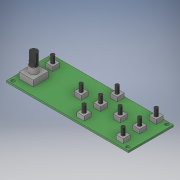
# Autodesk Inventor part: Keypad
Saved by Autodesk Inventor 2018 (Build 220112000, 112)
## iProperties
Created: 2013-10-28
Part Number: Keypad
Material: Generic
Document SubType Name: Modeling
Designer: Gabriel Smolnycki
Mass: 8.54171 g
Surface Area: 100.523 cm^2
Volume: 8.54171 cm^3
Density: 1 g/cm^3
Appearance: Default
Sending System: SolidWorks 2017
Last Author: Gabriel Smolnycki
Last Saved: 2017-09-14
Author: Gabriel Smolnycki
Autodesk Inventor part; units mm, degrees
ref_plane "YZ Plane" through (0, 0, 0) normal (1, 0, 0) x (0, 1, 0)
ref_plane "XZ Plane" through (0, 0, 0) normal (0, 1, 0) x (-1, 0, 0)
ref_plane "XY Plane" through (0, 0, 0) normal (0, 0, 1) x (1, 0, 0)
sketch "Sketch1" plane through (0, 0, 0) normal (0, 1, 0) x (-1, 0, 0)
  line L0 (-51.5, -19) -> (51.5, -19)
  line L1 (-51.5, 19) -> (-51.5, -19)
  line L2 (51.5, 19) -> (-51.5, 19)
  line L3 (51.5, -19) -> (51.5, 19)
  constraints: 8 end point, 2 horizontal, 2 vertical
extrude "Extrusion23" add sketch "Sketch1" along normal blind 1.5
hole "Hole4" at (48.5, 0, -16.5) direction (0, 1, 0) diameter 3 depth 1.5
hole "Hole3" at (48.5, 0, 16.5) direction (0, 1, 0) diameter 3 depth 1.5
sketch "Sketch3" plane through (0, 0, 0) normal (0, 1, 0) x (-1, 0, 0)
  point P0 (-48.5, 16.5)
hole "Hole2" at (-48.5, 0, 16.5) direction (0, 1, 0) diameter 3 depth 1.5
sketch "Sketch2" plane through (0, 0, 0) normal (0, 1, 0) x (-1, 0, 0)
  point P0 (-48.5, -16.5)
hole "Hole1" at (-48.5, 0, -16.5) direction (0, 1, 0) diameter 3 depth 1.5
sketch "Sketch6" plane through (0, 1.5, 0) normal (0, 1, 0) x (1, 0, 0)
  line L0 (44, 18) -> (38, 18)
  line L1 (44, 12) -> (44, 18)
  line L2 (38, 12) -> (44, 12)
  line L3 (38, 18) -> (38, 12)
  constraints: 8 end point, 2 horizontal, 2 vertical, 1 perpendicular
extrude "Extrusion22" add sketch "Sketch6" along normal blind 3.5
sketch "Sketch7" plane through (0, 1.5, 0) normal (0, 1, 0) x (1, 0, 0)
  line L0 (38, 4) -> (38, -2)
  line L1 (44, 4) -> (38, 4)
  line L2 (44, -2) -> (44, 4)
  line L3 (38, -2) -> (44, -2)
  constraints: 8 end point, 2 horizontal, 2 vertical, 1 perpendicular
extrude "Extrusion21" add sketch "Sketch7" along normal blind 3.5
sketch "Sketch8" plane through (0, 1.5, 0) normal (0, 1, 0) x (1, 0, 0)
  line L0 (38, -16) -> (44, -16)
  line L1 (38, -10) -> (38, -16)
  line L2 (44, -10) -> (38, -10)
  line L3 (44, -16) -> (44, -10)
  constraints: 8 end point, 2 horizontal, 2 vertical, 1 perpendicular
extrude "Extrusion20" add sketch "Sketch8" along normal blind 3.5
sketch "Sketch9" plane through (0, 1.5, 0) normal (0, 1, 0) x (1, 0, 0)
  line L0 (27.5, -2) -> (27.5, 4)
  line L1 (21.5, -2) -> (27.5, -2)
  line L2 (27.5, 4) -> (21.5, 4)
  line L3 (21.5, 4) -> (21.5, -2)
  constraints: 8 end point, 2 horizontal, 2 vertical, 1 perpendicular
extrude "Extrusion19" add sketch "Sketch9" along normal blind 3.5
sketch "Sketch10" plane through (0, 1.5, 0) normal (0, 1, 0) x (1, 0, 0)
  line L0 (5, 18) -> (5, 12)
  line L1 (11, 18) -> (5, 18)
  line L2 (11, 12) -> (11, 18)
  line L3 (5, 12) -> (11, 12)
  constraints: 8 end point, 2 horizontal, 2 vertical, 1 perpendicular
extrude "Extrusion18" add sketch "Sketch10" along normal blind 3.5
sketch "Sketch11" plane through (0, 1.5, 0) normal (0, 1, 0) x (1, 0, 0)
  line L0 (11, -2) -> (11, 4)
  line L1 (5, -2) -> (11, -2)
  line L2 (5, 4) -> (5, -2)
  line L3 (11, 4) -> (5, 4)
  constraints: 8 end point, 2 horizontal, 2 vertical, 1 perpendicular
extrude "Extrusion17" add sketch "Sketch11" along normal blind 3.5
sketch "Sketch12" plane through (0, 1.5, 0) normal (0, 1, 0) x (1, 0, 0)
  line L0 (5, -16) -> (11, -16)
  line L1 (11, -16) -> (11, -10)
  line L2 (11, -10) -> (5, -10)
  line L3 (5, -10) -> (5, -16)
  constraints: 8 end point, 2 horizontal, 2 vertical, 1 perpendicular
extrude "Extrusion16" add sketch "Sketch12" along normal blind 3.5
sketch "Sketch13" plane through (0, 1.5, 0) normal (0, 1, 0) x (1, 0, 0)
  line L0 (-11.5, 4) -> (-11.5, -2)
  line L1 (-5.5, 4) -> (-11.5, 4)
  line L2 (-5.5, -2) -> (-5.5, 4)
  line L3 (-11.5, -2) -> (-5.5, -2)
  constraints: 8 end point, 2 horizontal, 2 vertical, 1 perpendicular
extrude "Extrusion15" add sketch "Sketch13" along normal blind 3.5
sketch "Sketch14" plane through (0, 1.5, 0) normal (0, 1, 0) x (1, 0, 0)
  line L0 (-44.5, 7) -> (-38.5, 7)
  line L1 (-44.5, 13) -> (-44.5, 7)
  line L2 (-38.5, 13) -> (-44.5, 13)
  line L3 (-38.5, 7) -> (-38.5, 13)
  constraints: 8 end point, 2 horizontal, 2 vertical, 1 perpendicular
extrude "Extrusion14" add sketch "Sketch14" along normal blind 3.5
sketch "Sketch15" plane through (0, 1.5, 0) normal (0, 1, 0) x (1, 0, 0)
  line L0 (-47.5, -12.5) -> (-35.5, -12.5)
  line L1 (-47.5, 0.5) -> (-47.5, -12.5)
  line L2 (-35.5, 0.5) -> (-47.5, 0.5)
  line L3 (-35.5, -12.5) -> (-35.5, 0.5)
  constraints: 8 end point, 2 horizontal, 2 vertical
extrude "Extrusion13" add sketch "Sketch15" along normal blind 5
sketch "Sketch16" plane through (0, 6.5, 0) normal (0, 1, 0) x (1, 0, 0)
  circle A0 centre (-41.5, -6) radius 3.5
  constraints: 1 centre point
extrude "Extrusion12" add sketch "Sketch16" along normal blind 5
sketch "Sketch17" plane through (0, 5, 0) normal (0, 1, 0) x (1, 0, 0)
  circle A0 centre (41, 15) radius 1.5
  constraints: 1 centre point
extrude "Extrusion11" add sketch "Sketch17" along normal blind 6
sketch "Sketch18" plane through (0, 5, 0) normal (0, 1, 0) x (1, 0, 0)
  circle A0 centre (41, 1) radius 1.5
  constraints: 1 centre point
extrude "Extrusion10" add sketch "Sketch18" along normal blind 6
sketch "Sketch19" plane through (0, 5, 0) normal (0, 1, 0) x (1, 0, 0)
  circle A0 centre (41, -13) radius 1.5
  constraints: 1 centre point
extrude "Extrusion9" add sketch "Sketch19" along normal blind 6
sketch "Sketch20" plane through (0, 5, 0) normal (0, 1, 0) x (1, 0, 0)
  circle A0 centre (24.5, 1) radius 1.5
  constraints: 1 centre point
extrude "Extrusion8" add sketch "Sketch20" along normal blind 6
sketch "Sketch21" plane through (0, 5, 0) normal (0, 1, 0) x (1, 0, 0)
  circle A0 centre (8, -13) radius 1.5
  constraints: 1 centre point
extrude "Extrusion7" add sketch "Sketch21" along normal blind 6
sketch "Sketch22" plane through (0, 5, 0) normal (0, 1, 0) x (1, 0, 0)
  circle A0 centre (8, 1) radius 1.5
  constraints: 1 centre point
extrude "Extrusion6" add sketch "Sketch22" along normal blind 6
sketch "Sketch23" plane through (0, 5, 0) normal (0, 1, 0) x (1, 0, 0)
  circle A0 centre (8, 15) radius 1.5
  constraints: 1 centre point
extrude "Extrusion5" add sketch "Sketch23" along normal blind 6
sketch "Sketch24" plane through (0, 5, 0) normal (0, 1, 0) x (1, 0, 0)
  circle A0 centre (-8.5, 1) radius 1.5
  constraints: 1 centre point
extrude "Extrusion4" add sketch "Sketch24" along normal blind 6
sketch "Sketch25" plane through (0, 5, 0) normal (0, 1, 0) x (1, 0, 0)
  circle A0 centre (-41.5, 10) radius 1.5
  constraints: 1 centre point
extrude "Extrusion3" add sketch "Sketch25" along normal blind 6
sketch "Sketch26" plane through (-41.5, 11.5, 6) normal (0, 1, 0) x (1, 0, 0)
  circle A0 centre (0, 0) radius 3
  constraints: 1 centre point
extrude "Extrusion2" add sketch "Sketch26" along normal blind 10
sketch "Sketch27" plane through (-41.5, 21.5, 6) normal (0, 1, 0) x (1, 0, 0)
  line L0 (-2.8284, -1) -> (2.8284, -1)
  arc A0 (-2.8284, -1) -> (2.8284, -1) centre (0, 0) ccw
  constraints: 2 end point, 2 point on circle, 1 centre point, 1 horizontal
extrude "Extrusion1" cut sketch "Sketch27" against normal blind 7
sketch "Sketch4" plane through (0, 0, 0) normal (0, 1, 0) x (-1, 0, 0)
  point P0 (48.5, 16.5)
sketch "Sketch5" plane through (0, 0, 0) normal (0, 1, 0) x (-1, 0, 0)
  point P0 (48.5, -16.5)
body "Solid3"
